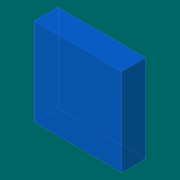
# Autodesk Inventor part: INFN Aerogel
Saved by Autodesk Inventor 2016 (Build 200138000, 138)
## iProperties
Created: 2016-02-03
Part Number: INFN Aerogel
Material: Glass
Document SubType Name: Modeling
Designer: Sawaiz
Density: 2.18 g/cm^3
Appearance: Clear - Blue
Author: Sawaiz
Autodesk Inventor part; units mm, degrees
ref_plane "YZ Plane" through (0, 0, 0) normal (1, 0, 0) x (0, 1, 0)
ref_plane "XZ Plane" through (0, 0, 0) normal (0, 1, 0) x (-1, 0, 0)
ref_plane "XY Plane" through (0, 0, 0) normal (0, 0, 1) x (1, 0, 0)
sketch "Sketch1" plane through (0, 0, 0) normal (1, 0, 0) x (0, 1, 0)
  line L0 (-55, -55) -> (55, -55)
  line L1 (55, -55) -> (55, 55)
  line L2 (55, 55) -> (-55, 55)
  line L3 (-55, 55) -> (-55, -55)
  line L4 (-55, -55) -> (55, 55) construction
  line L5 (55, -55) -> (-55, 55) construction
  point P0 (0, 0)
  dimension "d0" = 110
  dimension "d1" = 110
  constraints: 12 end point, 2 midpoint, 2 parallel, 1 horizontal, 1 perpendicular
  measures "d0" distance of L2.end L1.end
  measures "d1" distance of L1.end L0.end
extrude "Extrusion1" add sketch "Sketch1" along normal blind 30
equation "\"d0\" = aerogelWidth"
equation "\"d1\" = aerogelHeight"
equation "\"d2\" = aerogelThickness"
equation "\"plasticThickness\" = 6.35"
equation "\"aerogelThickness\" = 30"
equation "\"aerogelWidth\" = 110"
equation "\"aerogelHeight\" = 110"
equation "\"aerogelHolderDepth\" = 36.5125"
equation "\"height\" = 127"
equation "\"width\" = 127"
equation "\"depth\" = 114.3"
equation "\"mirrorAngle\" = 5deg"
equation "\"mirrorThickness\" = 3.175"
equation "\"fresnelThickness\" = 0.254"
equation "\"focalLength\" = 76.2"
equation "\"ior\" = 1.49"
equation "\"centerThickness\" = 1.27"
equation "\"fresnelAngle\" = 90deg"
equation "\"fresnelEffectiveDiameter\" = 152.4"
equation "\"caseThickness\" = 6.35"
equation "\"alignmentGrooveDepth\" = 1.5875"
equation "\"alignmentGrooveClearance\" = 0.1016"
equation "\"frontPanelThickness\" = 2.38125"
body "Solid1"
